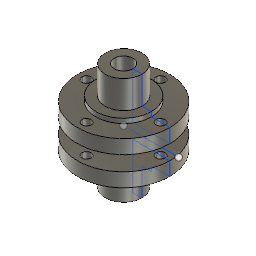
_Coupling Flange 1.aff28261-b530-4db2-8985-cc85df6f46d3 (Autodesk Fusion 360 design; units mm, degrees)
Autodesk Fusion 360 part; units mm, degrees
sketch "Sketch1" plane through (0, 0, 0) normal (0, 1, 0) x (1, 0, 0)
  line L0 (10, -60) -> (10, -10)
  line L1 (10, -10) -> (50, -10)
  line L2 (50, -10) -> (50, -25)
  line L3 (50, -25) -> (30, -25)
  line L4 (30, -25) -> (30, -30)
  line L5 (30, -30) -> (20, -30)
  line L6 (20, -30) -> (20, -60)
  line L7 (10, -60) -> (20, -60)
  line L8 (59.5256, -1.9963) -> (0, -1.9963)
  line L9 (10, 56.0073) -> (20, 56.0073)
  line L10 (20, 26.0073) -> (20, 56.0073)
  line L11 (10, 56.0073) -> (10, 6.0073)
  line L12 (10, 6.0073) -> (50, 6.0073)
  line L13 (50, 6.0073) -> (50, 21.0073)
  line L14 (50, 21.0073) -> (30, 21.0073)
  line L15 (30, 21.0073) -> (30, 26.0073)
  line L16 (30, 26.0073) -> (20, 26.0073)
revolve "Revolve2" add sketch "Sketch1" angle 360 about axis through (0, 0, 1.75) along (0, 0, 1) makes body 1 at (36.4433, -2.9808, 10) makes body 2 at (36.4433, -2.9808, -6.0073)
revolve "Revolve1" add sketch "Sketch1" angle 360 about axis through (0, 0, 1.75) along (0, 0, 1) separate body contours L0 L1 L2 L3 L4 L5 L6 L7 makes body 3
sketch "Sketch2" plane through (0, 0, 25) normal (0, 0, 1) x (-1, 0, 0)
  circle A0 centre (0, 0) radius 50
  circle A1 centre (0, 0) radius 30
  circle A2 centre (0, -40) radius 5
  circle A3 centre (-40, 0) radius 5
  circle A4 centre (0, 40) radius 5
  circle A5 centre (40, 0) radius 5
extrude "Extrude1" cut sketch "Sketch2" against normal blind 50 contours A2 | A3 | A4 | A5 bodies 1 2 3
